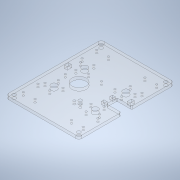
# Autodesk Inventor part: x-Axis_plate_bottom_t
Saved by Autodesk Inventor 2022 (Build 260153000, 153)
## iProperties
Created: 2021-04-15
Part Number: x-Axis_plate_bottom_t
Material: PET Plastic
Document SubType Name: Modeling
Designer: Fabijan_Sven
Density: 1.541 g/cm^3
Appearance: Polycarbonate - Clear
Mass: 161.085 g
Surface Area: 486.546 cm^2
Volume: 104.533 cm^3
Author: Fabijan_Sven
Autodesk Inventor part; units mm, degrees
ref_plane "YZ Plane" through (0, 0, 0) normal (1, 0, 0) x (0, 1, 0)
ref_plane "XZ Plane" through (0, 0, 0) normal (0, 1, 0) x (-1, 0, 0)
ref_plane "XY Plane" through (0, 0, 0) normal (0, 0, 1) x (1, 0, 0)
sketch "Sketch1" plane through (0, 0, 0) normal (0, 1, 0) x (-1, 0, 0)
  line L0 (0, 0) -> (124, 0)
  line L1 (124, 0) -> (124, -162)
  line L2 (124, -162) -> (0, -162)
  line L3 (0, -162) -> (0, 0)
  line L4 (117.9854, -81) -> (-11.1436, -81) construction
  line L5 (62, -11.2083) -> (62, -206.7638) construction
  circle A0 centre (113, -18.5) radius 1.6
  circle A1 centre (113, -43.5) radius 1.6
  circle A2 centre (93, -18.5) radius 1.6
  circle A3 centre (93, -43.5) radius 1.6
  circle A4 centre (113, -143.5) radius 1.6
  circle A5 centre (113, -118.5) radius 1.6
  circle A6 centre (93, -143.5) radius 1.6
  circle A7 centre (93, -118.5) radius 1.6
  circle A8 centre (11, -18.5) radius 1.6
  circle A9 centre (11, -43.5) radius 1.6
  circle A10 centre (31, -18.5) radius 1.6
  circle A11 centre (31, -43.5) radius 1.6
  circle A12 centre (11, -118.5) radius 1.6
  circle A13 centre (31, -143.5) radius 1.6
  circle A14 centre (11, -143.5) radius 1.6
  circle A15 centre (31, -118.5) radius 1.6
  line L6 (118, -93.5) -> (113, -93.5)
  line L7 (113, -93.5) -> (113, -100.5)
  line L8 (113, -100.5) -> (118, -100.5)
  line L9 (118, -100.5) -> (118, -93.5)
  line L10 (6, -93.5) -> (11, -93.5)
  line L11 (11, -93.5) -> (11, -100.5)
  line L12 (11, -100.5) -> (6, -100.5)
  line L13 (6, -100.5) -> (6, -93.5)
  circle A16 centre (7.5, -7.5) radius 2.8374
  circle A17 centre (37.5, -7.5) radius 2.5792
  circle A18 centre (7.5, -107.5) radius 2.9237
  circle A19 centre (37.5, -107.5) radius 2.6656
  dimension "d0" = 162
  dimension "d1" = 124
  dimension "d2" = 81
  dimension "d3" = 62
  dimension "d4" = 3.2
  dimension "d8" = 25
  dimension "d9" = 25
  dimension "d10" = 18.5
  dimension "d11" = 18.5
  dimension "d12" = 20
  dimension "d13" = 20
  dimension "d14" = 11
  dimension "d15" = 11
  dimension "d21" = 61.5
  dimension "d22" = 7
  dimension "d23" = 5
  dimension "d24" = 6
  dimension "d26" = 7.5
  dimension "d27" = 7.5
  dimension "d28" = 37.5
  dimension "d29" = 7.5
  dimension "d30" = 37.5
  dimension "d31" = 7.5
  dimension "d32" = 107.5
  dimension "d33" = 107.5
  constraints: 28 end point, 20 centre point, 16 symmetric about line, 4 parallel, 3 equal radius, 3 horizontal, 2 perpendicular, 1 vertical, 12 other
  measures "d0" distance of L0.end L1.end
  measures "d1" distance of L1.end L2.end
  measures "d2" distance between parallel lines of L0 L4
  measures "d3" distance between parallel lines of L1 L5
  measures "d4" diameter of A0
  measures "d8" distance of A0.centre A1.centre
  measures "d9" distance of A3.centre A2.centre
  measures "d10" distance from line of L0 A0.centre
  measures "d11" distance from line of L0 A2.centre
  measures "d12" distance of A2.centre A0.centre
  measures "d13" distance of A3.centre A1.centre
  measures "d14" distance from line of A0.centre L1
  measures "d15" distance from line of L1 A1.centre
  measures "d21" distance between parallel lines of L8 L2
  measures "d22" distance of L8.end L6.start
  measures "d23" distance of L6.start L6.end
  measures "d24" distance between parallel lines of L1 L9
  measures "d26" distance from line of L0 A17.centre
  measures "d27" distance from line of L0 A16.centre
  measures "d28" distance from line of L3 A17.centre
  measures "d29" distance from line of L3 A16.centre
  measures "d30" distance from line of L3 A19.centre
  measures "d31" distance from line of L3 A18.centre
  measures "d32" distance from line of A19.centre L0
  measures "d33" distance from line of L0 A18.centre
extrude "Extrusion1" add sketch "Sketch1" along normal blind 5 contours L0 L1 L2 L3 | A16 | A17 | A18 | A19
fillet "Fillet2" radius 5 4 edges at (0, 2.5, 0) (0, 2.5, -162) (-124, 2.5, -162) (-124, 2.5, 0)
sketch "Sketch3" plane through (0, 5, 0) normal (0, 1, 0) x (1, 0, 0)
  circle A0 centre (-93, 43.5) radius 1.8241
  line L0 (0, 5) -> (0, 157) projected
  circle A1 centre (-97, 54.8137) radius 5.6411
  circle A2 centre (-97, 54.8137) radius 16
  line L1 (-112.1751, 81) -> (15.1489, 81) construction
  line L2 (-119, 0) -> (-5, 0) projected
  circle A3 centre (-93, 118.5) radius 3.1
  circle A4 centre (-93, 118.5) radius 1.8241
  circle A5 centre (-97, 107.1863) radius 5.6411
  circle A6 centre (-97, 107.1863) radius 16
  circle A7 centre (-85.6863, 58.8137) radius 1.8241
  circle A8 centre (-101, 66.1274) radius 1.8241
  circle A9 centre (-108.3137, 50.8137) radius 1.8241
  circle A10 centre (-97, 54.8137) radius 5.6411
  circle A11 centre (-101, 95.8726) radius 1.8241
  circle A12 centre (-108.3137, 111.1863) radius 1.8241
  line L3 (-124, 157) -> (-124, 5) projected
  line L4 (-62, -8.3299) -> (-62, 205.5694) construction
  circle A13 centre (-31, 43.5) radius 3.1
  circle A14 centre (-31, 43.5) radius 1.8241
  circle A15 centre (-27, 54.8137) radius 5.6411
  circle A16 centre (-27, 54.8137) radius 16
  circle A17 centre (-31, 118.5) radius 3.1
  circle A18 centre (-31, 118.5) radius 1.8241
  circle A19 centre (-27, 107.1863) radius 5.6411
  circle A20 centre (-27, 107.1863) radius 16
  circle A21 centre (-38.3137, 58.8137) radius 1.8241
  circle A22 centre (-23, 66.1274) radius 1.8241
  circle A23 centre (-15.6863, 50.8137) radius 1.8241
  circle A24 centre (-27, 54.8137) radius 5.6411
  circle A25 centre (-15.6863, 111.1863) radius 1.8241
  circle A26 centre (-23, 95.8726) radius 1.8241
  circle A27 centre (-93, 43.5) radius 1.6 projected
  point P0 (0, 0)
  dimension "d57" = 12
  dimension "d59" = 32
  dimension "d60" = 81
  dimension "d63" = 360
  dimension "d66" = 62
  dimension "d89" = 124
  dimension "d200" = 0
  dimension "d201" = 0
  dimension "d202" = 70
  constraints: 27 centre point, 19 symmetric about line, 7 coincident, 4 end point, 1 horizontal, 1 vertical, 28 other
  measures "d57" distance of A1.centre A0.centre
  measures "d59" diameter of A2
  measures "d60" distance between parallel lines of L2 L1
  measures "d66" distance between parallel lines of L0 L4
  measures "d89" distance between parallel lines of L0 L3
  measures "d200" distance of A27.centre A0.centre
  measures "d201" distance of A27.centre A0.centre
  measures "d202" distance of A24.centre A2.centre
hole "Hole1" at (-108.3137, 5, -50.8137) at (-101, 5, -66.1274) at (-85.6863, 5, -58.8137) at (-108.3137, 5, -111.1863) at (-101, 5, -95.8726) at (-23, 5, -95.8726) at (-15.6863, 5, -111.1863) at (-38.3137, 5, -58.8137) at (-23, 5, -66.1274) at (-15.6863, 5, -50.8137) direction (0, -1, 0) diameter 3.2 end through all
sketch "Sketch4" plane through (0, 5, 0) normal (0, 1, 0) x (1, 0, 0)
  circle A0 centre (-97, 54.8137) radius 4
  circle A1 centre (-97, 107.1863) radius 4
  circle A2 centre (-27, 107.1863) radius 4 projected
  circle A3 centre (-27, 54.8137) radius 4 projected
  point P0 (0, 0)
  dimension "d203" = 70
  constraints: 2 centre point, 2 horizontal alignment, 1 vertical alignment
  measures "d203" distance of A3.centre A0.centre
hole "Hole2" at (-97, 5, -54.8137) at (-97, 5, -107.1863) at (-27, 5, -107.1863) at (-27, 5, -54.8137) direction (0, -1, 0) diameter 10 end through all
sketch "Sketch5" plane through (0, 5, 0) normal (0, 1, 0) x (1, 0, 0)
  circle A0 centre (-80.5, 81) radius 12
  line L0 (0, 5) -> (0, 157) projected
  line L1 (-119, 0) -> (-5, 0) projected
  circle A1 centre (-80.5, 81) radius 12 construction
  point P0 (0, 0)
  dimension "d81" = 24
  dimension "d82" = 80.5
  dimension "d83" = 81
  dimension "d90" = 24
  constraints: 2 centre point, 1 coincident
  measures "d81" diameter of A0
  measures "d82" distance from line of L0 A0.centre
  measures "d83" distance from line of L1 A0.centre
  measures "d90" diameter of A1
extrude "Extrusion3" cut sketch "Sketch5" against normal blind 2
sketch "Sketch6" plane through (-80.5, 3, -81) normal (0, 1, 0) x (1, 0, 0)
  circle A0 centre (0, 0) radius 12
  point P0 (80.5, -81)
  dimension "d86" = 24
  constraints: 1 centre point
  measures "d86" diameter of A0
extrude "Extrusion4" cut sketch "Sketch6" against normal blind 24
sketch "Sketch7" plane through (0, 5, 0) normal (0, 1, 0) x (1, 0, 0)
  circle A0 centre (-84.5, 101) radius 1.5
  line L0 (-124, 157) -> (-124, 5) projected
  circle A1 centre (-62.5, 101) radius 1.5
  circle A2 centre (-39.5, 101) radius 1.5
  line L1 (-5, 162) -> (-119, 162) projected
  point P0 (0, 0)
  point P1 (-92.5, 103)
  point P2 (-47.5, 103)
  point P3 (-70.5, 103)
  dimension "d190" = 3
  dimension "d191" = 39.5
  dimension "d192" = 3
  dimension "d193" = 3
  dimension "d194" = 84.5
  dimension "d195" = 61.5
  dimension "d196" = 61
  constraints: 3 centre point, 2 horizontal alignment
  measures "d190" diameter of A0
  measures "d191" distance from line of A0.centre L0
  measures "d192" diameter of A1
  measures "d193" diameter of A2
  measures "d194" distance from line of L0 A2.centre
  measures "d195" distance from line of L0 A1.centre
  measures "d196" distance from line of L1 A0.centre
hole "Hole3" at (-84.5, 5, -101) at (-62.5, 5, -101) at (-39.5, 5, -101) direction (0, -1, 0) diameter 3 end through all
sketch "Sketch8" plane through (0, 5, 0) normal (0, 1, 0) x (1, 0, 0)
  line L0 (-147.8175, 81) -> (38.0677, 81) construction
  line L1 (-62, -18.8902) -> (-62, 202.7642) construction
  line L2 (-5, 162) -> (-119, 162) projected
  line L3 (-119, 0) -> (-5, 0) projected
  line L4 (0, 5) -> (0, 157) projected
  line L5 (-124, 157) -> (-124, 5) projected
  circle A0 centre (-7, 7) radius 3
  circle A1 centre (-7, 155) radius 3
  circle A2 centre (-117, 7) radius 3
  circle A3 centre (-117, 155) radius 3
  point P0 (0, 0)
  dimension "d104" = 162
  dimension "d105" = 124
  dimension "d106" = 62
  dimension "d107" = 81
  dimension "d108" = 6
  dimension "d109" = 7
  dimension "d110" = 7
  constraints: 4 centre point, 4 end point, 3 symmetric about line, 1 horizontal, 1 vertical, 3 other
  measures "d104" distance between parallel lines of L2 L3
  measures "d105" distance between parallel lines of L4 L5
  measures "d106" distance between parallel lines of L1 L5
  measures "d107" distance between parallel lines of L2 L0
  measures "d108" diameter of A0
  measures "d109" distance from line of L4 A0.centre
  measures "d110" distance from line of A0.centre L3
hole "Hole4" at (-7, 5, -7) at (-117, 5, -7) at (-117, 5, -155) at (-7, 5, -155) direction (0, -1, 0) diameter 6 end through all
sketch "Sketch10" plane through (0, 5, 0) normal (0, 1, 0) x (1, 0, 0)
  line L0 (0, 5) -> (0, 157) projected
  line L1 (0, 72) -> (-25, 72)
  line L2 (-25, 72) -> (-25, 90)
  line L3 (-25, 90) -> (0, 90)
  line L4 (0, 90) -> (0, 72)
  line L5 (-119, 0) -> (-5, 0) projected
  line L6 (-33.2, 71.8) -> (-28, 71.8)
  line L7 (-28, 71.8) -> (-28, 76)
  line L8 (-28, 76) -> (-33.2, 76)
  line L9 (-33.2, 76) -> (-33.2, 71.8)
  line L10 (-33.2, 86) -> (-28, 86)
  line L11 (-28, 86) -> (-28, 90.2)
  line L12 (-28, 90.2) -> (-33.2, 90.2)
  line L13 (-33.2, 90.2) -> (-33.2, 86)
  point P0 (0, 0)
  point P1 (0, 90)
  dimension "d128" = 18
  dimension "d129" = 72
  dimension "d130" = 25
  dimension "d184" = 4.2
  dimension "d185" = 5.2
  dimension "d186" = 4.2
  dimension "d187" = 18.4
  dimension "d188" = 0.2
  dimension "d189" = 3
  constraints: 24 end point, 6 parallel, 3 horizontal, 3 perpendicular, 3 point on line
  measures "d128" distance of L1.end L2.end
  measures "d129" distance between parallel lines of L5 L1
  measures "d130" distance of L2.end L3.end
  measures "d184" distance between parallel lines of L8 L6
  measures "d185" distance between parallel lines of L7 L9
  measures "d186" distance between parallel lines of L12 L10
  measures "d187" distance between parallel lines of L12 L6
  measures "d188" distance between parallel lines of L1 L6
  measures "d189" distance between parallel lines of L2 L7
extrude "Extrusion5" cut sketch "Sketch10" against normal blind 10
fillet "Fillet4" radius 2 2 edges at (0, 2.5, -90) (0, 2.5, -72)
sketch "Sketch12" plane through (0, 0, 0) normal (0, -1, 0) x (1, 0, 0)
  circle A0 centre (-47, -49.5) radius 2
  circle A1 centre (-57, -49.5) radius 2
  line L0 (-119, 0) -> (-5, 0) projected
  line L1 (-40, -51) -> (-40, -46) projected
  circle A2 centre (-47, -49.5) radius 1.2295 projected
  circle A3 centre (-47, -49.5) radius 1.2295 projected
  circle A4 centre (-47, -49.5) radius 1.2295 projected
  circle A5 centre (-57, -49.5) radius 1.2295 projected
  point P0 (0, 0)
  dimension "d142" = 4
  dimension "d144" = 4
  constraints: 2 centre point, 2 concentric
  measures "d142" diameter of A0
  measures "d144" diameter of A1
hole "Hole7" at (-47, 0, -49.5) at (-57, 0, -49.5) direction (0, 1, 0) diameter 4 depth 20 tip angle 118
sketch "Sketch13" plane through (0, 5, 0) normal (0, 1, 0) x (1, 0, 0)
  circle A0 centre (-104, 81) radius 1.5
  line L0 (-124, 157) -> (-124, 5) projected
  line L1 (-119, 0) -> (-5, 0) projected
  point P0 (0, 0)
  dimension "d154" = 3
  dimension "d155" = 20
  dimension "d156" = 81
  constraints: 1 centre point
  measures "d154" diameter of A0
  measures "d155" distance from line of L0 A0.centre
  measures "d156" distance from line of L1 A0.centre
hole "Hole8" at (-104, 5, -81) direction (0, -1, 0) diameter 3.2 depth 20 tip angle 118
sketch "Sketch14" plane through (0, 5, 0) normal (0, 1, 0) x (1, 0, 0)
  circle A0 centre (-52.5, 55) radius 3
  line L0 (-119, 0) -> (-5, 0) projected
  line L1 (0, 5) -> (0, 70) projected
  point P0 (0, 0)
  dimension "d164" = 55
  dimension "d165" = 52.5
  dimension "d166" = 6
  constraints: 1 centre point
  measures "d164" distance from line of A0.centre L0
  measures "d165" distance from line of L1 A0.centre
  measures "d166" diameter of A0
hole "Hole9" at (-52.5, 5, -55) direction (0, -1, 0) diameter 6 depth 20 tip angle 118
fillet "Fillet6" radius 1.5 2 edges at (-25, 2.5, -72) (-25, 2.5, -90)
equation "\"d2\" = 0.5 * d0"
equation "\"d3\" = 0.5 * d1"
equation "\"d66\" = 0.5 * d89"
equation "\"d106\" = 0.5 * d105"
equation "\"d107\" = 0.5 * d104"
equation "\"d147\" = d144"
equation "\"d167\" = d166"
body "Solid1"
